# Autodesk Inventor part: SERIAL_MOLEX-1X4
Saved by Autodesk Inventor 2013 (Build 170138000, 138)
## iProperties
Created: 2014-11-03
Part Number: SERIAL_MOLEX-1X4
Material: Generic
Document SubType Name: Modeling
Designer: Jeramy
Density: 1 g/cm^3
Author: Jeramy
Autodesk Inventor part; units mm, degrees
ref_plane "YZ Plane" through (0, 0, 0) normal (1, 0, 0) x (0, 1, 0)
ref_plane "XZ Plane" through (0, 0, 0) normal (0, 1, 0) x (-1, 0, 0)
ref_plane "XY Plane" through (0, 0, 0) normal (0, 0, 1) x (1, 0, 0)
sketch "MOLEX-1X4, SERIAL_MOLEX-1X4_3" plane through (0, 0, 0) normal (0, 0, 1) x (1, 0, 0)
  line L0 (-1.3335, 3.1115) -> (8.89, 3.1115)
  line L1 (8.89, 3.1115) -> (8.89, -2.6035)
  line L2 (8.89, -2.6035) -> (-1.3335, -2.6035)
  line L3 (-1.3335, -2.6035) -> (-1.3335, 3.1115)
  constraints: 8 end point
extrude "Extrusion1" add sketch "MOLEX-1X4, SERIAL_MOLEX-1X4_3" along normal blind 1
body "Solid1"
